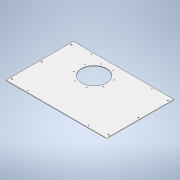
# Autodesk Inventor part: RearPanel
Saved by Autodesk Inventor 2020 (Build 240168000, 168)
## iProperties
Created: 2019-11-09
Part Number: RearPanel
Material: Generic
Document SubType Name: Modeling
Designer: nicoc
Density: 1 g/cm^3
Appearance: Default
Author: nicoc
Autodesk Inventor part; units mm, degrees
ref_plane "YZ Plane" through (0, 0, 0) normal (1, 0, 0) x (0, 1, 0)
ref_plane "XZ Plane" through (0, 0, 0) normal (0, 1, 0) x (-1, 0, 0)
ref_plane "XY Plane" through (0, 0, 0) normal (0, 0, 1) x (1, 0, 0)
sketch "Sketch1" plane through (0, 0, 0) normal (0, 1, 0) x (-1, 0, 0)
  line L0 (0, 0) -> (1000, 0)
  line L1 (1000, 0) -> (1000, -669)
  line L2 (1000, -669) -> (0, -669)
  line L3 (0, -669) -> (0, 0)
  dimension "d0" = 1000
  dimension "d1" = 669
  constraints: 8 end point, 2 parallel, 1 horizontal, 1 perpendicular
  measures "d0" distance between parallel lines of L1 L3
  measures "d1" distance between parallel lines of L2 L0
extrude "Extrusion1" add sketch "Sketch1" along normal blind 5
sketch "Sketch2" plane through (0, 5, 0) normal (0, 1, 0) x (1, 0, 0)
  circle A0 centre (-600, 475) radius 125
  line L0 (-1000, 0) -> (0, 0) projected
  line L1 (0, 0) -> (0, 669) projected
  dimension "d4" = 250
  dimension "d5" = 475
  dimension "d6" = 600
  constraints: 1 centre point
  measures "d4" diameter of A0
  measures "d5" distance from line of A0.centre L0
  measures "d6" distance from line of L1 A0.centre
extrude "Extrusion2" cut sketch "Sketch2" against normal through all
sketch "Sketch3" plane through (0, 5, 0) normal (0, 1, 0) x (1, 0, 0)
  line L0 (0, 0) -> (0, 669) projected
  line L1 (-1000, 0) -> (0, 0) projected
  line L2 (0, 669) -> (-1000, 669) projected
  line L3 (-1000, 669) -> (-1000, 0) projected
  point P0 (-20, 40)
  point P1 (-20, 335)
  point P2 (-20, 629)
  point P3 (-980, 40)
  point P4 (-980, 335)
  point P5 (-980, 629)
  dimension "d9" = 20
  dimension "d11" = 40
  dimension "d12" = 335
  dimension "d13" = 20
  dimension "d14" = 40
  dimension "d15" = 20
  dimension "d16" = 40
  dimension "d17" = 20
  dimension "d18" = 335
  dimension "d19" = 20
  dimension "d20" = 20
  dimension "d21" = 40
  measures "d9" distance from line of point (-20, 40) L0
  measures "d11" distance from line of point (-20, 40) L1
  measures "d12" distance from line of L1 point (-20, 335)
  measures "d13" distance from line of L0 point (-20, 335)
  measures "d14" distance from line of point (-20, 629) L2
  measures "d15" distance from line of L0 point (-20, 629)
  measures "d16" distance from line of point (-980, 40) L1
  measures "d17" distance from line of L3 point (-980, 40)
  measures "d18" distance from line of L1 point (-980, 335)
  measures "d19" distance from line of L3 point (-980, 335)
  measures "d20" distance from line of L3 point (-980, 629)
  measures "d21" distance from line of L2 point (-980, 629)
hole "Hole1" at (-20, 5, -40) at (-20, 5, -335) at (-20, 5, -629) at (-980, 5, -40) at (-980, 5, -335) at (-980, 5, -629) direction (0, -1, 0) diameter 5.5 end through all countersink diameter 11.5 countersink angle 90
sketch "Sketch5" plane through (0, 5, 0) normal (0, 1, 0) x (1, 0, 0)
  point P0 (0, 0)
sketch "Sketch6" plane through (0, 5, 0) normal (0, 1, 0) x (1, 0, 0)
  line L0 (-1000, 0) -> (0, 0) projected
  line L1 (0, 0) -> (0, 669) projected
  circle A0 centre (-600, 475) radius 125 projected
  point P0 (-650, 333.5786)
  dimension "d48" = 650
  dimension "d49" = 150
  measures "d48" distance from line of L1 point (-650, 333.579)
  measures "d49" distance of A0.centre point (-650, 333.579)
hole "Hole3" at (-650, 5, -333.5786) direction (0, -1, 0) diameter 6.647 end through all thread size "M8x1.25" class "6H" standard "ISO Metric profile"
pattern_circular "Circular Pattern1" count 8 over 360 about axis through (-600, 5, -475) along (0, -1, 0) of "Hole3"
sketch "Sketch7" plane through (0, 5, 0) normal (0, 1, 0) x (1, 0, 0)
  line L0 (-1000, 0) -> (0, 0) projected
  line L1 (0, 0) -> (0, 669) projected
  line L2 (0, 669) -> (-1000, 669) projected
  point P0 (-800, 19.5)
  point P1 (-800, 649.5)
  dimension "d54" = 19.5
  dimension "d55" = 800
  dimension "d56" = 800
  dimension "d68" = 19.5
  measures "d54" distance from line of point (-800, 19.5) L0
  measures "d55" distance from line of point (-800, 649.5) L1
  measures "d56" distance from line of L1 point (-800, 19.5)
  measures "d68" distance from line of L2 point (-800, 649.5)
hole "Hole4" at (-800, 5, -649.5) at (-800, 5, -19.5) direction (0, -1, 0) diameter 6.647 end through all thread size "M8x1.25" class "6H" standard "ISO Metric profile"
sketch "Sketch8" plane through (0, 5, 0) normal (0, 1, 0) x (1, 0, 0)
  line L0 (-1000, 0) -> (0, 0) projected
  line L1 (0, 0) -> (0, 669) projected
  line L2 (0, 669) -> (-1000, 669) projected
  point P0 (-200, 19.5)
  point P1 (-200, 649.5)
  dimension "d80" = 19.5
  dimension "d81" = 200
  dimension "d82" = 200
  dimension "d83" = 19.5
  measures "d80" distance from line of L0 point (-200, 19.5)
  measures "d81" distance from line of point (-200, 19.5) L1
  measures "d82" distance from line of point (-200, 649.5) L1
  measures "d83" distance from line of L2 point (-200, 649.5)
hole "Hole5" at (-200, 5, -19.5) at (-200, 5, -649.5) direction (0, -1, 0) diameter 6.647 end through all thread size "M8x1.25" class "6H" standard "ISO Metric profile"
equation "\"d13\" = d9"
equation "\"d14\" = d11"
equation "\"d15\" = d9"
equation "\"d16\" = d11"
equation "\"d17\" = d9"
equation "\"d18\" = d12"
equation "\"d19\" = d9"
equation "\"d20\" = d9"
equation "\"d21\" = d11"
equation "\"d55\" = d56"
equation "\"d68\" = d54"
equation "\"d82\" = d81"
equation "\"d83\" = d80"
body "Solid1"
